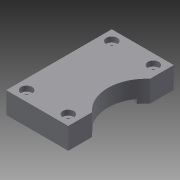
# Autodesk Inventor part: AdjusterSmallTop
Saved by Autodesk Inventor 2015 (Build 190159000, 159)
## iProperties
Created: 2017-01-31
Part Number: AdjusterSmallTop
Material: Generic
Document SubType Name: Modeling
Designer: Ernest
Density: 1 g/cm^3
Appearance: Default
Author: Ernest
Autodesk Inventor part; units mm, degrees
ref_plane "YZ Plane" through (0, 0, 0) normal (1, 0, 0) x (0, 1, 0)
ref_plane "XZ Plane" through (0, 0, 0) normal (0, 1, 0) x (-1, 0, 0)
ref_plane "XY Plane" through (0, 0, 0) normal (0, 0, 1) x (1, 0, 0)
sketch "Sketch1" plane through (0, 0, 0) normal (0, 1, 0) x (-1, 0, 0)
  arc A0 (-20.4235, 23.3213) -> (20.4235, 23.3213) centre (0, 0) ccw
  line L0 (0, 0) -> (0, 31) construction
  arc A1 (-16.9701, 14.7738) -> (16.9701, 14.7738) centre (0, 0) ccw
  arc A2 (-18.2123, 17.8484) -> (18.2123, 17.8484) centre (0, 0) ccw
  line L1 (0, 0) -> (-11.6128, 28.7427)
  line L2 (0, 0) -> (11.6128, 28.7427)
  line L3 (-22.9815, 43) -> (-13.0218, 18.3489)
  line L4 (-6.6269, 30.2834) -> (-3.3791, 22.2448)
  line L5 (6.6269, 30.2834) -> (3.3791, 22.2448)
  line L6 (22.9815, 43) -> (13.0218, 18.3489)
  circle A3 centre (0, 0) radius 38
  line L7 (-16.9701, 14.7738) -> (-23.1699, 30.119)
  line L8 (23.1699, 30.119) -> (16.9701, 14.7738)
  line L9 (-23.1699, 30.119) -> (-23.1699, 43)
  line L10 (-23.1699, 43) -> (23.1699, 43)
  line L11 (23.1699, 43) -> (23.1699, 30.119)
  arc A4 (-13.0218, 18.3489) -> (-16.9701, 14.7738) centre (0, 0) ccw
  arc A5 (16.9701, 14.7738) -> (13.0218, 18.3489) centre (0, 0) ccw
  arc A6 (-8.4286, 20.8616) -> (-13.0218, 18.3489) centre (0, 0) ccw
  arc A7 (0, 22.5) -> (-8.4286, 20.8616) centre (0, 0) ccw
  arc A8 (3.3791, 22.2448) -> (0, 22.5) centre (0, 0) ccw
  arc A9 (8.4286, 20.8616) -> (3.3791, 22.2448) centre (0, 0) ccw
  arc A10 (13.0218, 18.3489) -> (8.4286, 20.8616) centre (0, 0) ccw
  arc A11 (-14.1731, 21.1984) -> (-18.2123, 17.8484) centre (0, 0) ccw
  arc A12 (-9.5525, 23.6432) -> (-14.1731, 21.1984) centre (0, 0) ccw
  arc A13 (-4.5304, 25.0943) -> (-9.5525, 23.6432) centre (0, 0) ccw
  arc A14 (0, 25.5) -> (-4.5304, 25.0943) centre (0, 0) ccw
  arc A15 (4.5304, 25.0943) -> (0, 25.5) centre (0, 0) ccw
  arc A16 (9.5525, 23.6432) -> (4.5304, 25.0943) centre (0, 0) ccw
  arc A17 (14.1731, 21.1984) -> (9.5525, 23.6432) centre (0, 0) ccw
  arc A18 (18.2123, 17.8484) -> (14.1731, 21.1984) centre (0, 0) ccw
  arc A19 (-16.2696, 26.3875) -> (-20.4235, 23.3213) centre (0, 0) ccw
  arc A20 (-11.6128, 28.7427) -> (-16.2696, 26.3875) centre (0, 0) ccw
  arc A21 (-6.6269, 30.2834) -> (-11.6128, 28.7427) centre (0, 0) ccw
  arc A22 (0, 31) -> (-6.6269, 30.2834) centre (0, 0) ccw
  arc A23 (6.6269, 30.2834) -> (0, 31) centre (0, 0) ccw
  arc A24 (11.6128, 28.7427) -> (6.6269, 30.2834) centre (0, 0) ccw
  arc A25 (16.2696, 26.3875) -> (11.6128, 28.7427) centre (0, 0) ccw
  arc A26 (20.4235, 23.3213) -> (16.2696, 26.3875) centre (0, 0) ccw
  point P0 (-18.9225, 32.9536)
  point P1 (18.9225, 32.9536)
  dimension "d2" = 62
  dimension "d46" = 10.4
  dimension "d47" = 10.4
  dimension "d48" = 5.2
  dimension "d49" = 5.2
  dimension "d50" = 22
  dimension "d51" = 22
  dimension "d52" = 76
  dimension "d53" = 5
  dimension "d54" = 5
  dimension "d55" = 5
  constraints: 82 point on circle, 27 centre point, 24 end point, 20 point on line, 6 parallel, 4 coincident, 2 perpendicular, 2 vertical
  measures "d2" diameter of A0
  measures "d46" distance between parallel lines of L4 L3
  measures "d47" distance between parallel lines of L6 L5
  measures "d48" distance between parallel lines of L2 L5
  measures "d49" distance between parallel lines of L1 L3
  measures "d50" angle of L0 L1
  measures "d51" angle of L0 L2
  measures "d52" diameter of A3
  measures "d53" distance between parallel lines of L3 L7
  measures "d54" distance between parallel lines of L6 L8
  measures "d55" distance edge to line of A3 L10
extrude "Extrusion11" add sketch "Sketch1" along normal blind 4 contours A19 L3 A11 L7 | L7 A3 L3 A19 | A26 L6 A3 L8 | L8 A18 L6 A26 | A11 L3 A4 L7 | L9 L10 L3 A3 | A20 L1 A12 L3 | L3 A3 L6 A25 A24 A23 A22 A21 A20 | A3 L6 L10 L11 | L8 A5 L6 A18 | L6 A17 L2 A25 | A12 L1 A6 L3 | L3 L10 L6 A3 | A21 L4 A13 L1 | L6 A10 L2 A17 | L2 A16 L5 A24 | A13 L4 A7 L1 | A22 A23 L5 A15 A14 L4 | L2 A9 L5 A16 | A14 A15 L5 A8 A7 L4
extrude "Extrusion12" add sketch "Sketch1" against normal blind 6 contours A19 L3 A11 L7 | L7 A3 L3 A19 | A26 L6 A3 L8 | L8 A18 L6 A26 | A11 L3 A4 L7 | L9 L10 L3 A3 | A20 L1 A12 L3 | A3 L6 L10 L11 | L8 A5 L6 A18 | L6 A17 L2 A25 | A12 L1 A6 L3 | L3 L10 L6 A3 | A21 L4 A13 L1 | L6 A10 L2 A17 | L2 A16 L5 A24 | A13 L4 A7 L1 | A22 A23 L5 A15 A14 L4 | L2 A9 L5 A16 | A14 A15 L5 A8 A7 L4
extrude "Extrusion13" add sketch "Sketch1" against normal blind 16.6 contours A19 L3 A11 L7 | L7 A3 L3 A19 | A26 L6 A3 L8 | L8 A18 L6 A26 | A11 L3 A4 L7 | L9 L10 L3 A3 | A3 L6 L10 L11 | L8 A5 L6 A18
sketch "Sketch8" plane through (0, -16.6, 0) normal (0, -1, 0) x (1, 0, 0)
  line L0 (22.9815, 43) -> (13.0218, 18.3489) projected
  arc A0 (16.9701, 14.7738) -> (13.0218, 18.3489) centre (0, 0) ccw projected
  line L1 (16.9701, 14.7738) -> (23.1699, 30.119) projected
  line L2 (23.1699, 30.119) -> (23.1699, 43) projected
  line L3 (23.1699, 43) -> (22.9815, 43) projected
  line L4 (18.9225, 32.9536) -> (22.9815, 43) projected
  line L5 (22.9815, 43) -> (-22.9815, 43) projected
  line L6 (-22.9815, 43) -> (-18.9225, 32.9536) projected
  arc A1 (18.9225, 32.9536) -> (-18.9225, 32.9536) centre (0, 0) ccw projected
  line L7 (-13.0218, 18.3489) -> (-22.9815, 43) projected
  line L8 (-22.9815, 43) -> (-23.1699, 43) projected
  line L9 (-23.1699, 43) -> (-23.1699, 30.119) projected
  line L10 (-23.1699, 30.119) -> (-16.9701, 14.7738) projected
  arc A2 (-13.0218, 18.3489) -> (-16.9701, 14.7738) centre (0, 0) ccw projected
  line L11 (16.9701, 14.7738) -> (27.1699, 14.7738)
  line L12 (27.1699, 14.7738) -> (27.1699, 49.8908)
  line L13 (27.1699, 49.8908) -> (-31.1699, 49.8908)
  line L14 (-31.1699, 49.8908) -> (-31.1699, 14.7738)
  line L15 (-31.1699, 14.7738) -> (-16.9701, 14.7738)
  line L16 (16.9701, 14.7738) -> (23.1699, 30.119)
  line L17 (23.1699, 30.119) -> (23.1699, 43)
  line L18 (-23.1699, 43) -> (-23.1699, 30.119)
  line L19 (-23.1699, 30.119) -> (-16.9701, 14.7738)
  line L20 (-22.9815, 43) -> (-18.9225, 32.9536) projected
  arc A3 (18.9225, 32.9536) -> (-18.9225, 32.9536) centre (0, 0) ccw projected
  arc A4 (23.1699, 43) -> (-23.1699, 43) centre (0, 0) ccw
  line L21 (23.1699, 43) -> (22.9815, 43)
  line L22 (-22.9815, 43) -> (-23.1699, 43)
  line L23 (18.9225, 32.9536) -> (-18.9225, 32.9536) construction
  line L24 (18.3165, 31.4536) -> (-18.3165, 31.4536)
  line L25 (19.5285, 34.4536) -> (-19.5285, 34.4536)
  line L26 (-11.3093, 41.8727) -> (-4.6215, 25.3198)
  line L27 (11.3094, 41.8729) -> (4.907, 26.0264)
  dimension "d62" = 8
  dimension "d63" = 4
  dimension "d64" = 3
  dimension "d65" = 1.5
  dimension "d66" = 10.4
  dimension "d68" = 10.4
  constraints: 34 end point, 8 parallel, 7 point on line, 4 perpendicular, 3 horizontal, 3 point on circle, 1 centre point, 1 coincident, 1 collinear, 1 vertical
  measures "d62" distance between parallel lines of L9 L14
  measures "d63" distance between parallel lines of L2 L12
  measures "d64" distance between parallel lines of L24 L25
  measures "d65" distance between parallel lines of L23 L25
  measures "d66" distance between parallel lines of L7 L26
  measures "d68" distance between parallel lines of L0 L27
sketch "Sketch9" plane through (0, -6, 0) normal (0, -1, 0) x (1, 0, 0)
  line L0 (18.9225, 32.9536) -> (22.9815, 43) projected
  line L1 (22.9815, 43) -> (-22.9815, 43) projected
  line L2 (-22.9815, 43) -> (-18.9225, 32.9536) projected
  arc A0 (18.9225, 32.9536) -> (-18.9225, 32.9536) centre (0, 0) ccw projected
extrude "Extrusion14" add sketch "Sketch9" along normal blind 2.6
sketch "Sketch10" plane through (0, -8.6, 0) normal (0, -1, 0) x (1, 0, 0)
  line L0 (22.9815, 43) -> (18.9225, 32.9536) projected
  line L1 (22.9815, 43) -> (-22.9815, 43) projected
  line L2 (-18.9225, 32.9536) -> (-22.9815, 43) projected
  arc A0 (18.9225, 32.9536) -> (-18.9225, 32.9536) centre (0, 0) ccw projected
  circle A1 centre (0, 0) radius 46
  line L3 (-23.1699, 43) -> (23.1699, 43) projected
  line L4 (16.3401, 43) -> (-16.3401, 43)
  line L5 (23.1699, 51.1984) -> (-23.1699, 51.1984)
  line L6 (-23.1699, 51.1984) -> (-23.1699, 43)
  line L7 (-23.1699, 43) -> (-16.3401, 43)
  line L8 (23.1699, 43) -> (23.1699, 51.1984)
  line L9 (23.1699, 43) -> (16.3401, 43)
  line L10 (23.1699, 43) -> (22.9815, 43) projected
  line L11 (22.9815, 43) -> (21.9428, 40.4291)
  line L12 (22.9815, 43) -> (18.9225, 32.9536) projected
  line L13 (-22.9815, 43) -> (-21.9428, 40.4291)
  line L14 (-18.9225, 32.9536) -> (-22.9815, 43) projected
  dimension "d71" = 92
  constraints: 16 end point, 4 point on circle, 4 point on line, 3 perpendicular, 1 centre point, 1 coincident, 1 collinear
  measures "d71" diameter of A1
extrude "Extrusion15" add sketch "Sketch10" against normal blind 12.6 contours L1 A1 L3 L6 L5 L8 | L1 A1
extrude "Extrusion16" add sketch "Sketch10" along normal blind 8 contours L0 A1 L1 | L1 A1 L3 L6 L5 L8 | A1 L2 L1
sketch "Sketch11" plane through (0, -16.6, 0) normal (0, -1, 0) x (1, 0, 0)
  line L0 (-13.0218, 18.3489) -> (-21.9428, 40.4291) projected
  arc A0 (21.9428, 40.4291) -> (-21.9428, 40.4291) centre (0, 0) ccw projected
  line L1 (21.9428, 40.4291) -> (13.0218, 18.3489) projected
  arc A1 (16.9701, 14.7738) -> (13.0218, 18.3489) centre (0, 0) ccw projected
  line L2 (16.9701, 14.7738) -> (23.1699, 30.119) projected
  line L3 (23.1699, 30.119) -> (23.1699, 51.1984) projected
  line L4 (23.1699, 51.1984) -> (-23.1699, 51.1984) projected
  line L5 (-23.1699, 51.1984) -> (-23.1699, 30.119) projected
  line L6 (-23.1699, 30.119) -> (-16.9701, 14.7738) projected
  arc A2 (-13.0218, 18.3489) -> (-16.9701, 14.7738) centre (0, 0) ccw projected
  arc A3 (18.9225, 32.9536) -> (-18.9225, 32.9536) centre (0, 0) ccw projected
  line L7 (-18.9225, 32.9536) -> (-16.2696, 26.3875) projected
  arc A4 (16.2696, 26.3875) -> (-16.2696, 26.3875) centre (0, 0) ccw projected
  line L8 (16.2696, 26.3875) -> (18.9225, 32.9536) projected
  line L9 (18.9225, 32.9536) -> (-18.9225, 32.9536) construction
  line L10 (-16.9701, 14.7738) -> (-30.9701, 14.7738)
  line L11 (-30.9701, 14.7738) -> (-30.9701, 51.1984)
  line L12 (-30.9701, 51.1984) -> (-23.1699, 51.1984)
  line L13 (-23.1699, 51.1984) -> (-23.1699, 30.119)
  line L14 (-23.1699, 30.119) -> (-16.9701, 14.7738)
  line L15 (-16.9701, 14.7738) -> (-23.1699, 30.119) projected
  line L16 (16.9701, 14.7738) -> (30.9701, 14.7738)
  line L17 (30.9701, 14.7738) -> (30.9701, 51.1984)
  line L18 (30.9701, 51.1984) -> (23.1699, 51.1984)
  line L19 (23.1699, 51.1984) -> (23.1699, 30.119)
  line L20 (23.1699, 30.119) -> (16.9701, 14.7738)
  line L21 (23.1699, 30.119) -> (16.9701, 14.7738) projected
  dimension "d76" = 14
  dimension "d88" = 14
  constraints: 22 end point, 4 perpendicular, 3 collinear, 3 horizontal, 1 vertical
  measures "d76" distance of L6.end L10.end
  measures "d88" distance of L2.start L16.end
extrude "Extrusion17" add sketch "Sketch11" against normal blind 20.6 contours L10 L11 L12 L5 L6 | L2 L3 L18 L17 L16
ref_plane "Work Plane2" through (0, -16.6, 14.7738) normal (-1, 0, 0) x (0, 0, 1)
sketch "Sketch12" plane through (0, -16.6, 14.7738) normal (-1, 0, 0) x (0, 0, 1)
  line L0 (25.6553, 0) -> (25.6553, 8) projected
  line L1 (25.6553, 8) -> (18.1797, 8) projected
  line L2 (18.1797, 16.6) -> (18.1797, 8) projected
  line L3 (11.6136, 16.6) -> (18.1797, 16.6) projected
  line L4 (11.6136, 10.6) -> (11.6136, 16.6) projected
  line L5 (3.5751, 10.6) -> (11.6136, 10.6) projected
  line L6 (3.5751, 10.6) -> (3.5751, 0) projected
  line L7 (25.6553, 0) -> (3.5751, 0) projected
  circle A0 centre (18.1797, 4) radius 1.65
  line L8 (25.6553, 0) -> (14.8797, 0)
  line L9 (14.8797, 0) -> (14.8797, 8)
  line L10 (14.8797, 8) -> (25.6553, 8)
  line L11 (25.6553, 8) -> (25.6553, 0)
  circle A1 centre (18.1797, 4) radius 2.6
  point P0 (-14.7738, 16.6)
  dimension "d79" = 3.3
  dimension "d80" = 3.3
  dimension "d83" = 5.2
  constraints: 8 end point, 2 centre point, 2 parallel, 1 coincident, 1 horizontal, 1 perpendicular, 1 point on line
  measures "d79" diameter of A0
  measures "d80" distance from line of L9 A0.centre
  measures "d83" diameter of A1
extrude "Extrusion18" cut sketch "Sketch12" along normal mid plane 62.85 contours A0
extrude "Extrusion19" cut sketch "Sketch12" along normal blind 24.1 contours A1
extrude "Extrusion20" cut sketch "Sketch12" against normal blind 24.1 contours L7 L9 L10 L1 L0 | A1
sketch "Sketch13" plane through (0, -16.6, 0) normal (0, -1, 0) x (1, 0, 0)
  line L0 (21.9428, 40.4291) -> (24.1, 40.4291) projected
  line L1 (24.1, 40.4291) -> (24.1, 29.6536) projected
  line L2 (24.1, 29.6536) -> (17.5892, 29.6536) projected
  line L3 (17.5892, 29.6536) -> (13.0218, 18.3489) projected
  arc A0 (16.9701, 14.7738) -> (13.0218, 18.3489) centre (0, 0) ccw projected
  line L4 (16.9701, 14.7738) -> (30.9701, 14.7738) projected
  line L5 (30.9701, 14.7738) -> (30.9701, 51.1984) projected
  line L6 (30.9701, 51.1984) -> (-30.9701, 51.1984) projected
  line L7 (-30.9701, 51.1984) -> (-30.9701, 14.7738) projected
  line L8 (-30.9701, 14.7738) -> (-16.9701, 14.7738) projected
  arc A1 (-13.0218, 18.3489) -> (-16.9701, 14.7738) centre (0, 0) ccw projected
  line L9 (-13.0218, 18.3489) -> (-21.9428, 40.4291) projected
  arc A2 (21.9428, 40.4291) -> (-21.9428, 40.4291) centre (0, 0) ccw projected
  circle A3 centre (24.9701, 20.7738) radius 1.5
  circle A4 centre (-24.9701, 20.7738) radius 1.5
  circle A5 centre (-24.9701, 45.1984) radius 1.5
  circle A6 centre (24.9701, 45.1984) radius 1.5
  dimension "d89" = 3
  dimension "d90" = 6
  dimension "d91" = 6
  dimension "d92" = 6
  dimension "d93" = 6
  dimension "d94" = 3
  dimension "d95" = 3
  dimension "d96" = 6
  dimension "d97" = 6
  dimension "d98" = 6
  dimension "d99" = 6
  dimension "d100" = 3
  constraints: 4 centre point
  measures "d89" diameter of A4
  measures "d90" distance from line of L5 A3.centre
  measures "d91" distance from line of L4 A3.centre
  measures "d92" distance from line of L7 A4.centre
  measures "d93" distance from line of L8 A4.centre
  measures "d94" diameter of A5
  measures "d95" diameter of A6
  measures "d96" distance from line of L5 A6.centre
  measures "d97" distance from line of L6 A6.centre
  measures "d98" distance from line of L7 A5.centre
  measures "d99" distance from line of L6 A5.centre
  measures "d100" diameter of A3
extrude "Extrusion21" cut sketch "Sketch13" against normal blind 33.6 contours A3 | A4 | A5 | A6
sketch "Sketch14" plane through (0, -16.6, 0) normal (0, -1, 0) x (1, 0, 0)
  circle A0 centre (-24.9701, 45.1984) radius 1.5 projected
  circle A1 centre (24.9701, 20.7738) radius 1.5 projected
  circle A2 centre (-24.9701, 20.7738) radius 1.5 projected
  circle A3 centre (24.9701, 45.1984) radius 1.5 projected
  line L0 (21.9428, 40.4291) -> (24.1, 40.4291) projected
  line L1 (24.1, 40.4291) -> (24.1, 29.6536) projected
  line L2 (24.1, 29.6536) -> (17.5892, 29.6536) projected
  line L3 (17.5892, 29.6536) -> (13.0218, 18.3489) projected
  arc A4 (16.9701, 14.7738) -> (13.0218, 18.3489) centre (0, 0) ccw projected
  line L4 (16.9701, 14.7738) -> (30.9701, 14.7738) projected
  line L5 (30.9701, 14.7738) -> (30.9701, 51.1984) projected
  line L6 (30.9701, 51.1984) -> (-30.9701, 51.1984) projected
  line L7 (-30.9701, 51.1984) -> (-30.9701, 14.7738) projected
  line L8 (-30.9701, 14.7738) -> (-16.9701, 14.7738) projected
  arc A5 (-13.0218, 18.3489) -> (-16.9701, 14.7738) centre (0, 0) ccw projected
  line L9 (-13.0218, 18.3489) -> (-21.9428, 40.4291) projected
  arc A6 (21.9428, 40.4291) -> (-21.9428, 40.4291) centre (0, 0) ccw projected
extrude "Extrusion22" cut sketch "Sketch14" against normal blind 8
sketch "Sketch15" plane through (0, 4, 0) normal (0, 1, 0) x (1, 0, 0)
  circle A0 centre (-24.9701, -45.1984) radius 1.5 projected
  circle A1 centre (24.9701, -20.7738) radius 1.5 projected
  circle A2 centre (-24.9701, -20.7738) radius 1.5 projected
  circle A3 centre (24.9701, -45.1984) radius 1.5 projected
  line L0 (-16.9701, -14.7738) -> (-30.9701, -14.7738) projected
  line L1 (-30.9701, -14.7738) -> (-30.9701, -51.1984) projected
  line L2 (-30.9701, -51.1984) -> (30.9701, -51.1984) projected
  line L3 (30.9701, -51.1984) -> (30.9701, -14.7738) projected
  line L4 (30.9701, -14.7738) -> (16.9701, -14.7738) projected
  arc A4 (-16.9701, -14.7738) -> (16.9701, -14.7738) centre (0, 0) ccw projected
  circle A5 centre (24.9701, -45.1984) radius 3.25
  circle A6 centre (24.9701, -20.7738) radius 3.25
  circle A7 centre (-24.9701, -45.1984) radius 1.5 projected
  circle A8 centre (-24.9701, -45.1984) radius 3.25
  circle A9 centre (-24.9701, -20.7738) radius 3.25
  dimension "d105" = 6.5
  dimension "d106" = 6.5
  dimension "d107" = 6.5
  dimension "d108" = 6.5
  constraints: 4 centre point, 4 coincident
  measures "d105" diameter of A5
  measures "d106" diameter of A6
  measures "d107" diameter of A8
  measures "d108" diameter of A9
extrude "Extrusion23" cut sketch "Sketch15" against normal blind 3 contours A5 | A6 | A8 | A9
equation "\"d51\" = d50"
body "Solid2"
